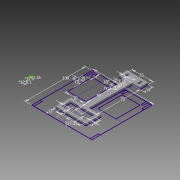
# Autodesk Inventor part: body-back
Saved by Autodesk Inventor 2013 (Build 170138000, 138)
## iProperties
Created: 2012-09-08
Part Number: body-back
Material: Generic
Document SubType Name: Modeling
Designer: frankenteddy
Density: 1 g/cm^3
Author: frankenteddy
Autodesk Inventor part; units mm, degrees
ref_plane "YZ Plane" through (0, 0, 0) normal (1, 0, 0) x (0, 1, 0)
ref_plane "XZ Plane" through (0, 0, 0) normal (0, 1, 0) x (-1, 0, 0)
ref_plane "XY Plane" through (0, 0, 0) normal (0, 0, 1) x (1, 0, 0)
sketch "Sketch1" plane through (0, 0, 0) normal (0, 0, 1) x (1, 0, 0)
  line L0 (-50, 50) -> (50, 50)
  line L1 (50, 50) -> (50, -50)
  line L2 (50, -50) -> (-50, -50)
  line L3 (-50, -50) -> (-50, 50)
  line L4 (-92.7646, -8.503) -> (-89.7646, -8.503)
  line L5 (-89.7646, -8.503) -> (-89.7646, -11.753)
  line L6 (-89.7646, -11.753) -> (-92.7646, -11.753)
  line L7 (-92.7646, -11.753) -> (-92.7646, -8.503)
  line L8 (-92.7646, -21.6527) -> (-89.7646, -21.6527)
  line L9 (-89.7646, -21.6527) -> (-89.7646, -21.7527)
  line L10 (-89.7646, -21.7527) -> (-92.7646, -21.7527)
  line L11 (-92.7646, -21.7527) -> (-92.7646, -21.6527)
  line L12 (-50, 50) -> (-46.75, 50)
  line L13 (-46.75, 50) -> (-46.75, 36)
  line L14 (-46.75, 36) -> (-50, 36)
  line L15 (-50, 36) -> (-50, 50)
  line L16 (0, 50) -> (0, -50) construction
  line L17 (-50, 0) -> (50, 0) construction
  line L18 (50, 50) -> (46.75, 50)
  line L19 (46.75, 50) -> (46.75, 36)
  line L20 (46.75, 36) -> (50, 36)
  line L21 (50, 36) -> (50, 50)
  line L22 (-50, -50) -> (-46.75, -50)
  line L23 (-46.75, -50) -> (-46.75, -36)
  line L24 (-46.75, -36) -> (-50, -36)
  line L25 (-50, -36) -> (-50, -50)
  line L26 (46.75, -50) -> (46.75, -36)
  line L27 (46.75, -36) -> (50, -36)
  line L28 (50, -36) -> (50, -50)
  line L29 (50, -50) -> (46.75, -50)
  line L30 (-40, 40) -> (-10, 40)
  line L31 (-10, 40) -> (-10, 0)
  line L32 (-10, 0) -> (-40, 0)
  line L33 (-40, 0) -> (-40, 40)
  line L34 (40, 40) -> (10, 40)
  line L35 (10, 40) -> (10, 0)
  line L36 (10, 0) -> (40, 0)
  line L37 (40, 0) -> (40, 40)
  line L38 (-10, 50) -> (-6.75, 50)
  line L39 (-6.75, 50) -> (-6.75, 42)
  line L40 (-6.75, 42) -> (-10, 42)
  line L41 (-10, 42) -> (-10, 50)
  line L42 (10, 50) -> (6.75, 50)
  line L43 (6.75, 50) -> (6.75, 42)
  line L44 (6.75, 42) -> (10, 42)
  line L45 (10, 42) -> (10, 50)
  line L46 (-25, 0) -> (-25, 40) construction
  line L47 (-40, 50) -> (-43.25, 50)
  line L48 (-43.25, 50) -> (-43.25, 42)
  line L49 (-43.25, 42) -> (-40, 42)
  line L50 (-40, 42) -> (-40, 50)
  line L51 (43.25, 42) -> (40, 42)
  line L52 (43.25, 50) -> (43.25, 42)
  line L53 (40, 50) -> (43.25, 50)
  line L54 (40, 42) -> (40, 50)
  line L55 (-20, -15) -> (20, -15)
  line L56 (20, -15) -> (20, -30)
  line L57 (20, -30) -> (-20, -30)
  line L58 (-20, -30) -> (-20, -15)
  line L59 (-25, -10) -> (25, -10)
  line L60 (25, -10) -> (25, -35)
  line L61 (25, -35) -> (-25, -35)
  line L62 (-25, -35) -> (-25, -10)
  line L63 (0, -15) -> (0, -30) construction
  line L64 (-5, -10) -> (5, -10)
  line L65 (5, -10) -> (5, 62)
  line L66 (5, 62) -> (-5, 62)
  line L67 (-5, 62) -> (-5, -10)
  line L68 (0, 62) -> (0, -10) construction
  line L69 (-17.5, 62) -> (17.5, 62)
  line L70 (17.5, 62) -> (17.5, 76)
  line L71 (17.5, 76) -> (-17.5, 76)
  line L72 (-17.5, 76) -> (-17.5, 62)
  line L73 (0, 76) -> (0, 62) construction
  line L74 (-20, -22.5) -> (20, -22.5) construction
  line L75 (-12.5, 72.5) -> (-9.25, 72.5)
  line L76 (-9.25, 72.5) -> (-9.25, 65.5)
  line L77 (-9.25, 65.5) -> (-12.5, 65.5)
  line L78 (-12.5, 65.5) -> (-12.5, 72.5)
  line L79 (-12.5, 69) -> (-9.25, 69) construction
  line L80 (12.5, 72.5) -> (9.25, 72.5)
  line L81 (9.25, 72.5) -> (9.25, 65.5)
  line L82 (9.25, 65.5) -> (12.5, 65.5)
  line L83 (12.5, 65.5) -> (12.5, 72.5)
  line L84 (12.5, 69) -> (9.25, 69) construction
  point P0 (0, 0)
  dimension "d0" = 100
  dimension "d2" = 100
  dimension "d3" = 3
  dimension "mat" = 3.25
  dimension "d5" = 3
  dimension "kerf" = 0.1
  dimension "d7" = 3.25
  dimension "d8" = 14
  dimension "d9" = 30
  dimension "d10" = 40
  dimension "d11" = 10
  dimension "d12" = 10
  dimension "d15" = 3.25
  dimension "d16" = 8
  dimension "d17" = 0
  dimension "d22" = 40
  dimension "d23" = 15
  dimension "d24" = 5
  dimension "d25" = 5
  dimension "d26" = 5
  dimension "d27" = 5
  dimension "d28" = 15
  dimension "d29" = 72
  dimension "d30" = 14
  dimension "d31" = 10
  dimension "d32" = 35
  dimension "d35" = 27.5
  dimension "d36" = 3.25
  dimension "d37" = 7
  dimension "d38" = 7
  dimension "d39" = 5
  constraints: 170 end point, 31 symmetric about line, 22 parallel, 18 midpoint, 11 horizontal, 11 perpendicular, 5 collinear, 1 point on line
  measures "d0" distance of L0.start L0.end
  measures "d2" distance of L2.end L0.start
  measures "d3" distance of L5.end L6.end
  measures "mat" distance of L4.end L5.end
  measures "d5" distance of L9.end L10.end
  measures "kerf" distance of L8.end L9.end
  measures "d7" distance of L13.end L14.end
  measures "d8" distance of L12.end L13.end
  measures "d9" distance of L31.end L32.end
  measures "d10" distance of L30.end L31.end
  measures "d11" distance between parallel lines of L30 L0
  measures "d12" distance between parallel lines of L3 L33
  measures "d15" distance of L39.end L40.end
  measures "d16" distance of L38.end L39.end
  measures "d17" distance between parallel lines of L41 L31
  measures "d22" distance of L56.end L57.end
  measures "d23" distance of L55.end L56.end
  measures "d24" distance between parallel lines of L59 L55
  measures "d25" distance between parallel lines of L58 L62
  measures "d26" distance between parallel lines of L61 L57
  measures "d27" distance between parallel lines of L60 L56
  measures "d28" distance between parallel lines of L2 L61
  measures "d29" distance of L64.end L65.end
  measures "d30" distance of L69.end L70.end
  measures "d31" distance of L64.start L64.end
  measures "d32" distance of L70.end L71.end
  measures "d35" distance between parallel lines of L2 L74
  measures "d36" distance of L76.end L77.end
  measures "d37" distance of L75.end L76.end
  measures "d38" distance between parallel lines of L69 L79
  measures "d39" distance between parallel lines of L72 L78
extrude "Extrusion4" add sketch "Sketch1" along normal blind 3.25 contours L67 L66 L65 L0 | L0 L65 L59 L67 | L69 L72 L71 L70 L66 | L59 L60 L61 L62 | L75 L76 L77 L78 | L83 L82 L81 L80
extrude "Extrusion5" cut sketch "Sketch1" along normal blind 3.25 contours L75 L76 L77 L78 | L83 L82 L81 L80
equation "\"d7\" = mat"
equation "\"d15\" = mat"
equation "\"d36\" = mat"
equation "\"d33\" = mat"
equation "\"d40\" = mat"
body "Solid2"
